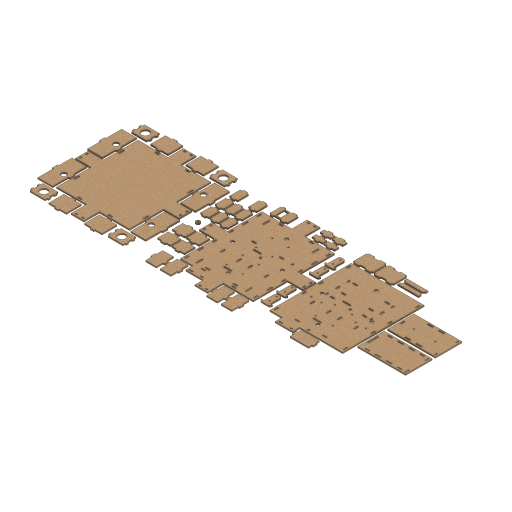
# Autodesk Inventor part: Pieza1
Saved by Autodesk Inventor 2024 (Build 280153000, 153)
## iProperties
Created: 2023-11-21
Part Number: Pieza1
Material: MDF Tablero de fibras de densidad media
Document SubType Name: Modeling
Designer: marco
Density: 0.8 g/cm^3
Appearance: Cartón - Ondulado
Author: marco
Autodesk Inventor part; units mm, degrees
(part 1 of 2)
ref_plane "YZ Plane" through (0, 0, 0) normal (1, 0, 0) x (0, 1, 0)
ref_plane "XZ Plane" through (0, 0, 0) normal (0, 1, 0) x (-1, 0, 0)
ref_plane "XY Plane" through (0, 0, 0) normal (0, 0, 1) x (1, 0, 0)
sketch "Boceto1" plane through (0, 0, 0) normal (0, 1, 0) x (-1, 0, 0)
  line L0 (397.5, 103.5) -> (397.5, 108.5)
  line L1 (397.5, 108.5) -> (400.5, 108.5)
  line L2 (400.5, 108.5) -> (400.5, 113.5)
  line L3 (400.5, 113.5) -> (397.5, 113.5)
  line L4 (397.5, 113.5) -> (397.5, 123.5)
  line L5 (397.5, 123.5) -> (400.5, 123.5)
  line L6 (400.5, 123.5) -> (400.5, 128.5)
  line L7 (400.5, 128.5) -> (397.5, 128.5)
  line L8 (397.5, 128.5) -> (397.5, 133.5)
  line L9 (397.5, 133.5) -> (362.5, 133.5)
  line L10 (362.5, 133.5) -> (362.5, 128.5)
  line L11 (362.5, 128.5) -> (359.5, 128.5)
  line L12 (359.5, 128.5) -> (359.5, 123.5)
  line L13 (359.5, 123.5) -> (362.5, 123.5)
  line L14 (362.5, 123.5) -> (362.5, 113.5)
  line L15 (362.5, 113.5) -> (359.5, 113.5)
  line L16 (359.5, 113.5) -> (359.5, 108.5)
  line L17 (359.5, 108.5) -> (362.5, 108.5)
  line L18 (362.5, 108.5) -> (362.5, 103.5)
  line L19 (362.5, 103.5) -> (397.5, 103.5)
  line L20 (180.5, 133.5) -> (180.5, 128.5)
  line L21 (180.5, 128.5) -> (177.5, 128.5)
  line L22 (177.5, 128.5) -> (177.5, 123.5)
  line L23 (177.5, 123.5) -> (180.5, 123.5)
  line L24 (180.5, 123.5) -> (180.5, 113.5)
  line L25 (180.5, 113.5) -> (177.5, 113.5)
  line L26 (177.5, 113.5) -> (177.5, 108.5)
  line L27 (177.5, 108.5) -> (180.5, 108.5)
  line L28 (180.5, 108.5) -> (180.5, 103.5)
  line L29 (180.5, 103.5) -> (215.5, 103.5)
  line L30 (215.5, 103.5) -> (215.5, 108.5)
  line L31 (215.5, 108.5) -> (218.5, 108.5)
  line L32 (218.5, 108.5) -> (218.5, 113.5)
  line L33 (218.5, 113.5) -> (215.5, 113.5)
  line L34 (215.5, 113.5) -> (215.5, 123.5)
  line L35 (215.5, 123.5) -> (218.5, 123.5)
  line L36 (218.5, 123.5) -> (218.5, 128.5)
  line L37 (218.5, 128.5) -> (215.5, 128.5)
  line L38 (215.5, 128.5) -> (215.5, 133.5)
  line L39 (215.5, 133.5) -> (180.5, 133.5)
  line L40 (329, -92) -> (320, -92)
  line L41 (320, -92) -> (320, -89)
  line L42 (320, -89) -> (329, -89)
  line L43 (329, -89) -> (329, -92)
  line L44 (371, 58) -> (368, 58)
  line L45 (368, 58) -> (368, 46)
  line L46 (368, 46) -> (371, 46)
  line L47 (371, 46) -> (371, 58)
  line L48 (320, 92) -> (329, 92)
  line L49 (329, 92) -> (329, 89)
  line L50 (329, 89) -> (320, 89)
  line L51 (320, 89) -> (320, 92)
  line L52 (371, -46) -> (368, -46)
  line L53 (368, -46) -> (368, -58)
  line L54 (368, -58) -> (371, -58)
  line L55 (371, -58) -> (371, -46)
  line L56 (207, -46) -> (210, -46)
  line L57 (210, -46) -> (210, -58)
  line L58 (210, -58) -> (207, -58)
  line L59 (207, -58) -> (207, -46)
  line L60 (174, -10) -> (171, -10)
  line L61 (171, -10) -> (171, -5)
  line L62 (171, -5) -> (174, -5)
  line L63 (174, -5) -> (174, -10)
  line L64 (207, 46) -> (210, 46)
  line L65 (210, 46) -> (210, 58)
  line L66 (210, 58) -> (207, 58)
  line L67 (207, 58) -> (207, 46)
  line L68 (258, -92) -> (249, -92)
  line L69 (249, -92) -> (249, -89)
  line L70 (249, -89) -> (258, -89)
  line L71 (258, -89) -> (258, -92)
  line L72 (279, -128) -> (279, -125)
  line L73 (279, -125) -> (284, -125)
  line L74 (284, -125) -> (284, -128)
  line L75 (284, -128) -> (279, -128)
  line L76 (299, 125) -> (294, 125)
  line L77 (294, 125) -> (294, 128)
  line L78 (294, 128) -> (299, 128)
  line L79 (299, 128) -> (299, 125)
  line L80 (284, 128) -> (279, 128)
  line L81 (279, 128) -> (279, 125)
  line L82 (279, 125) -> (284, 125)
  line L83 (284, 125) -> (284, 128)
  line L84 (404, -10) -> (404, -5)
  line L85 (404, -5) -> (407, -5)
  line L86 (407, -5) -> (407, -10)
  line L87 (407, -10) -> (404, -10)
  line L88 (404, 5) -> (404, 10)
  line L89 (404, 10) -> (407, 10)
  line L90 (407, 10) -> (407, 5)
  line L91 (407, 5) -> (404, 5)
  line L92 (299, -125) -> (294, -125)
  line L93 (294, -125) -> (294, -128)
  line L94 (294, -128) -> (299, -128)
  line L95 (299, -128) -> (299, -125)
  line L96 (174, 10) -> (174, 5)
  line L97 (174, 5) -> (171, 5)
  line L98 (171, 5) -> (171, 10)
  line L99 (171, 10) -> (174, 10)
  line L100 (415, -49) -> (418, -49)
  line L101 (418, -49) -> (418, -61)
  line L102 (418, -61) -> (415, -61)
  line L103 (415, -61) -> (415, -98)
  line L104 (415, -98) -> (380, -98)
  line L105 (380, -98) -> (380, -61)
  line L106 (380, -61) -> (377, -61)
  line L107 (377, -61) -> (377, -49)
  line L108 (377, -49) -> (380, -49)
  line L109 (380, -49) -> (380, -18)
  line L110 (380, -18) -> (415, -18)
  line L111 (415, -18) -> (415, -49)
  line L112 (377, 49) -> (377, 61)
  line L113 (377, 61) -> (380, 61)
  line L114 (380, 61) -> (380, 98)
  line L115 (380, 98) -> (415, 98)
  line L116 (415, 98) -> (415, 61)
  line L117 (415, 61) -> (418, 61)
  line L118 (418, 61) -> (418, 49)
  line L119 (418, 49) -> (415, 49)
  line L120 (415, 49) -> (415, 18)
  line L121 (415, 18) -> (380, 18)
  line L122 (380, 18) -> (380, 49)
  line L123 (380, 49) -> (377, 49)
  line L124 (163, 98) -> (198, 98)
  line L125 (198, 98) -> (198, 61)
  line L126 (198, 61) -> (201, 61)
  line L127 (201, 61) -> (201, 49)
  line L128 (201, 49) -> (198, 49)
  line L129 (198, 49) -> (198, 18)
  line L130 (198, 18) -> (163, 18)
  line L131 (163, 18) -> (163, 49)
  line L132 (163, 49) -> (160, 49)
  line L133 (160, 49) -> (160, 61)
  line L134 (160, 61) -> (163, 61)
  line L135 (163, 61) -> (163, 98)
  line L136 (258, 92) -> (249, 92)
  line L137 (249, 92) -> (249, 89)
  line L138 (249, 89) -> (258, 89)
  line L139 (258, 89) -> (258, 92)
  line L140 (310, 101) -> (310, 136)
  line L141 (310, 136) -> (326, 136)
  line L142 (326, 136) -> (326, 139)
  line L143 (326, 139) -> (335, 139)
  line L144 (335, 139) -> (335, 136)
  line L145 (335, 136) -> (351, 136)
  line L146 (351, 136) -> (351, 101)
  line L147 (351, 101) -> (335, 101)
  line L148 (335, 101) -> (335, 98)
  line L149 (335, 98) -> (326, 98)
  line L150 (326, 98) -> (326, 101)
  line L151 (326, 101) -> (310, 101)
  line L152 (310, -136) -> (310, -101)
  line L153 (310, -101) -> (326, -101)
  line L154 (326, -101) -> (326, -98)
  line L155 (326, -98) -> (335, -98)
  line L156 (335, -98) -> (335, -101)
  line L157 (335, -101) -> (351, -101)
  line L158 (351, -101) -> (351, -136)
  line L159 (351, -136) -> (335, -136)
  line L160 (335, -136) -> (335, -139)
  line L161 (335, -139) -> (326, -139)
  line L162 (326, -139) -> (326, -136)
  line L163 (326, -136) -> (310, -136)
  line L164 (362.5, -133.5) -> (397.5, -133.5)
  line L165 (397.5, -133.5) -> (397.5, -128.5)
  line L166 (397.5, -128.5) -> (400.5, -128.5)
  line L167 (400.5, -128.5) -> (400.5, -123.5)
  line L168 (400.5, -123.5) -> (397.5, -123.5)
  line L169 (397.5, -123.5) -> (397.5, -113.5)
  line L170 (397.5, -113.5) -> (400.5, -113.5)
  line L171 (400.5, -113.5) -> (400.5, -108.5)
  line L172 (400.5, -108.5) -> (397.5, -108.5)
  line L173 (397.5, -108.5) -> (397.5, -103.5)
  line L174 (397.5, -103.5) -> (362.5, -103.5)
  line L175 (362.5, -103.5) -> (362.5, -108.5)
  line L176 (362.5, -108.5) -> (359.5, -108.5)
  line L177 (359.5, -108.5) -> (359.5, -113.5)
  line L178 (359.5, -113.5) -> (362.5, -113.5)
  line L179 (362.5, -113.5) -> (362.5, -123.5)
  line L180 (362.5, -123.5) -> (359.5, -123.5)
  line L181 (359.5, -123.5) -> (359.5, -128.5)
  line L182 (359.5, -128.5) -> (362.5, -128.5)
  line L183 (362.5, -128.5) -> (362.5, -133.5)
  line L184 (177.5, -123.5) -> (177.5, -128.5)
  line L185 (177.5, -128.5) -> (180.5, -128.5)
  line L186 (180.5, -128.5) -> (180.5, -133.5)
  line L187 (180.5, -133.5) -> (215.5, -133.5)
  line L188 (215.5, -133.5) -> (215.5, -128.5)
  line L189 (215.5, -128.5) -> (218.5, -128.5)
  line L190 (218.5, -128.5) -> (218.5, -123.5)
  line L191 (218.5, -123.5) -> (215.5, -123.5)
  line L192 (215.5, -123.5) -> (215.5, -113.5)
  line L193 (215.5, -113.5) -> (218.5, -113.5)
  line L194 (218.5, -113.5) -> (218.5, -108.5)
  line L195 (218.5, -108.5) -> (215.5, -108.5)
  line L196 (215.5, -108.5) -> (215.5, -103.5)
  line L197 (215.5, -103.5) -> (180.5, -103.5)
  line L198 (180.5, -103.5) -> (180.5, -108.5)
  line L199 (180.5, -108.5) -> (177.5, -108.5)
  line L200 (177.5, -108.5) -> (177.5, -113.5)
  line L201 (177.5, -113.5) -> (180.5, -113.5)
  line L202 (180.5, -113.5) -> (180.5, -123.5)
  line L203 (180.5, -123.5) -> (177.5, -123.5)
  line L204 (138.7318, -1.5139) -> (136.2318, -1.5139)
  line L205 (136.2318, -1.5139) -> (136.2318, 1.4861)
  line L206 (136.2318, 1.4861) -> (141.2318, 1.4861)
  line L207 (141.2318, 1.4861) -> (141.2318, -1.5139)
  line L208 (141.2318, -1.5139) -> (138.7318, -1.5139)
  line L209 (-20.6092, 99.402) -> (-20.6092, 114.402)
  line L210 (-20.6092, 114.402) -> (-17.6092, 114.402)
  line L211 (-17.6092, 114.402) -> (-17.6092, 124.402)
  line L212 (-17.6092, 124.402) -> (-20.6092, 124.402)
  line L213 (-20.6092, 124.402) -> (-20.6092, 139.402)
  line L214 (-20.6092, 139.402) -> (-45.6092, 139.402)
  line L215 (-45.6092, 139.402) -> (-45.6092, 124.402)
  line L216 (-45.6092, 124.402) -> (-48.6092, 124.402)
  line L217 (-48.6092, 124.402) -> (-48.6092, 114.402)
  line L218 (-48.6092, 114.402) -> (-45.6092, 114.402)
  line L219 (-45.6092, 114.402) -> (-45.6092, 99.402)
  line L220 (-45.6092, 99.402) -> (-20.6092, 99.402)
  line L221 (45.6946, -98.4202) -> (36.6946, -98.4202)
  line L222 (36.6946, -98.4202) -> (36.6946, -101.4202)
  line L223 (36.6946, -101.4202) -> (31.6946, -101.4202)
  line L224 (31.6946, -101.4202) -> (31.6946, -126.4202)
  line L225 (31.6946, -126.4202) -> (36.6946, -126.4202)
  line L226 (36.6946, -126.4202) -> (36.6946, -129.4202)
  line L227 (36.6946, -129.4202) -> (45.6946, -129.4202)
  line L228 (45.6946, -129.4202) -> (45.6946, -126.4202)
  line L229 (45.6946, -126.4202) -> (63.1946, -126.4202)
  line L230 (63.1946, -126.4202) -> (63.1946, -129.4202)
  line L231 (63.1946, -129.4202) -> (69.1946, -129.4202)
  line L232 (69.1946, -98.4202) -> (63.1946, -98.4202)
  line L233 (63.1946, -98.4202) -> (63.1946, -101.4202)
  line L234 (63.1946, -101.4202) -> (45.6946, -101.4202)
  line L235 (45.6946, -101.4202) -> (45.6946, -98.4202)
  line L236 (-54.5593, 99.402) -> (-54.5593, 114.402)
  line L237 (-54.5593, 114.402) -> (-51.5593, 114.402)
  line L238 (-51.5593, 114.402) -> (-51.5593, 124.402)
  line L239 (-51.5593, 124.402) -> (-54.5593, 124.402)
  line L240 (-54.5593, 124.402) -> (-54.5593, 139.402)
  line L241 (-54.5593, 139.402) -> (-79.5593, 139.402)
  line L242 (-79.5593, 139.402) -> (-79.5593, 124.402)
  line L243 (-79.5593, 124.402) -> (-82.5593, 124.402)
  line L244 (-82.5593, 124.402) -> (-82.5593, 114.402)
  line L245 (-82.5593, 114.402) -> (-79.5593, 114.402)
  line L246 (-79.5593, 114.402) -> (-79.5593, 99.402)
  line L247 (-79.5593, 99.402) -> (-54.5593, 99.402)
  line L248 (121.6406, 99.402) -> (121.6406, 114.402)
  line L249 (121.6406, 114.402) -> (124.6406, 114.402)
  line L250 (124.6406, 114.402) -> (124.6406, 124.402)
  line L251 (124.6406, 124.402) -> (121.6406, 124.402)
  line L252 (121.6406, 124.402) -> (121.6406, 139.402)
  line L253 (121.6406, 139.402) -> (96.6406, 139.402)
  line L254 (96.6406, 139.402) -> (96.6406, 124.402)
  line L255 (96.6406, 124.402) -> (93.6406, 124.402)
  line L256 (93.6406, 124.402) -> (93.6406, 114.402)
  line L257 (93.6406, 114.402) -> (96.6406, 114.402)
  line L258 (96.6406, 114.402) -> (96.6406, 99.402)
  line L259 (96.6406, 99.402) -> (121.6406, 99.402)
  line L260 (87.6406, 99.402) -> (87.6406, 114.402)
  line L261 (87.6406, 114.402) -> (90.6406, 114.402)
  line L262 (90.6406, 114.402) -> (90.6406, 124.402)
  line L263 (90.6406, 124.402) -> (87.6406, 124.402)
  line L264 (87.6406, 124.402) -> (87.6406, 139.402)
  line L265 (87.6406, 139.402) -> (62.6406, 139.402)
  line L266 (62.6406, 139.402) -> (62.6406, 124.402)
  line L267 (62.6406, 124.402) -> (59.6406, 124.402)
  line L268 (59.6406, 124.402) -> (59.6406, 114.402)
  line L269 (59.6406, 114.402) -> (62.6406, 114.402)
  line L270 (62.6406, 114.402) -> (62.6406, 99.402)
  line L271 (62.6406, 99.402) -> (87.6406, 99.402)
  line L272 (-24.9127, -131.1401) -> (-32.4127, -131.1401)
  line L273 (-32.4127, -131.1401) -> (-32.4127, -134.1401)
  line L274 (-32.4127, -134.1401) -> (-42.4127, -134.1401)
  line L275 (-42.4127, -134.1401) -> (-42.4127, -131.1401)
  line L276 (-42.4127, -131.1401) -> (-49.9127, -131.1401)
  line L277 (-49.9127, -131.1401) -> (-49.9127, -121.1401)
  line L278 (-49.9127, -121.1401) -> (-42.4127, -121.1401)
  line L279 (-42.4127, -121.1401) -> (-42.4127, -118.1401)
  line L280 (-42.4127, -118.1401) -> (-32.4127, -118.1401)
  line L281 (-32.4127, -118.1401) -> (-32.4127, -121.1401)
  line L282 (-32.4127, -121.1401) -> (-24.9127, -121.1401)
  line L283 (-24.9127, -121.1401) -> (-24.9127, -131.1401)
  line L284 (-387.9327, 9.6476) -> (-397.9327, 9.6476)
  line L285 (-397.9327, 9.6476) -> (-397.9327, 6.6476)
  line L286 (-397.9327, 6.6476) -> (-387.9327, 6.6476)
  line L287 (-387.9327, 6.6476) -> (-387.9327, 9.6476)
  line L288 (-411.4327, 3.6476) -> (-299.4327, 3.6476)
  line L289 (-299.4327, 3.6476) -> (-299.4327, 65.6476)
  line L290 (-299.4327, 65.6476) -> (-411.4327, 65.6476)
  line L291 (-411.4327, 65.6476) -> (-411.4327, 3.6476)
  line L292 (-322.9327, 59.6476) -> (-322.9327, 62.6476)
  line L293 (-322.9327, 62.6476) -> (-312.9327, 62.6476)
  line L294 (-312.9327, 62.6476) -> (-312.9327, 59.6476)
  line L295 (-312.9327, 59.6476) -> (-322.9327, 59.6476)
  line L296 (-322.9327, 9.6476) -> (-322.9327, 6.6476)
  line L297 (-322.9327, 6.6476) -> (-312.9327, 6.6476)
  line L298 (-312.9327, 6.6476) -> (-312.9327, 9.6476)
  line L299 (-312.9327, 9.6476) -> (-322.9327, 9.6476)
  line L300 (-312.9327, 9.6476) -> (-322.9327, 9.6476)
  line L301 (-322.9327, 9.6476) -> (-322.9327, 6.6476)
  line L302 (-322.9327, 6.6476) -> (-312.9327, 6.6476)
  line L303 (-312.9327, 6.6476) -> (-312.9327, 9.6476)
  line L304 (-397.9327, 59.6476) -> (-387.9327, 59.6476)
  line L305 (-387.9327, 59.6476) -> (-387.9327, 62.6476)
  line L306 (-387.9327, 62.6476) -> (-397.9327, 62.6476)
  line L307 (-397.9327, 62.6476) -> (-397.9327, 59.6476)
  line L308 (-335.9327, 6.6476) -> (-348.9327, 6.6476)
  line L309 (-348.9327, 6.6476) -> (-348.9327, 9.6476)
  line L310 (-348.9327, 9.6476) -> (-335.9327, 9.6476)
  line L311 (-335.9327, 9.6476) -> (-335.9327, 6.6476)
  line L312 (-361.9327, 6.6476) -> (-374.9327, 6.6476)
  line L313 (-374.9327, 6.6476) -> (-374.9327, 9.6476)
  line L314 (-374.9327, 9.6476) -> (-361.9327, 9.6476)
  line L315 (-361.9327, 9.6476) -> (-361.9327, 6.6476)
  line L316 (-335.9327, 62.6476) -> (-335.9327, 59.6476)
  line L317 (-335.9327, 59.6476) -> (-348.9327, 59.6476)
  line L318 (-348.9327, 59.6476) -> (-348.9327, 62.6476)
  line L319 (-348.9327, 62.6476) -> (-335.9327, 62.6476)
  line L320 (-361.9327, 62.6476) -> (-361.9327, 59.6476)
  line L321 (-361.9327, 59.6476) -> (-374.9327, 59.6476)
  line L322 (-374.9327, 59.6476) -> (-374.9327, 62.6476)
  line L323 (-374.9327, 62.6476) -> (-361.9327, 62.6476)
  line L324 (-60.4127, -134.1401) -> (-60.4127, -131.1401)
  line L325 (-60.4127, -131.1401) -> (-52.9127, -131.1401)
  line L326 (-52.9127, -131.1401) -> (-52.9127, -121.1401)
  line L327 (-52.9127, -121.1401) -> (-60.4127, -121.1401)
  line L328 (-60.4127, -121.1401) -> (-60.4127, -118.1401)
  line L329 (-60.4127, -118.1401) -> (-70.4127, -118.1401)
  line L330 (-70.4127, -118.1401) -> (-70.4127, -121.1401)
  line L331 (-70.4127, -121.1401) -> (-77.9127, -121.1401)
  line L332 (-77.9127, -121.1401) -> (-77.9127, -131.1401)
  line L333 (-77.9127, -131.1401) -> (-70.4127, -131.1401)
  line L334 (-70.4127, -131.1401) -> (-70.4127, -134.1401)
  line L335 (-70.4127, -134.1401) -> (-60.4127, -134.1401)
  line L336 (-77.9127, -102.1401) -> (-77.9127, -112.1401)
  line L337 (-77.9127, -112.1401) -> (-70.4127, -112.1401)
  line L338 (-70.4127, -112.1401) -> (-70.4127, -115.1401)
  line L339 (-70.4127, -115.1401) -> (-60.4127, -115.1401)
  line L340 (-60.4127, -115.1401) -> (-60.4127, -112.1401)
  line L341 (-60.4127, -112.1401) -> (-52.9127, -112.1401)
  line L342 (-52.9127, -112.1401) -> (-52.9127, -102.1401)
  line L343 (-52.9127, -102.1401) -> (-60.4127, -102.1401)
  line L344 (-60.4127, -102.1401) -> (-60.4127, -99.1401)
  line L345 (-60.4127, -99.1401) -> (-70.4127, -99.1401)
  line L346 (-70.4127, -99.1401) -> (-70.4127, -102.1401)
  line L347 (-70.4127, -102.1401) -> (-77.9127, -102.1401)
  line L348 (-32.4127, -115.1401) -> (-32.4127, -112.1401)
  line L349 (-32.4127, -112.1401) -> (-24.9127, -112.1401)
  line L350 (-24.9127, -112.1401) -> (-24.9127, -102.1401)
  line L351 (-24.9127, -102.1401) -> (-32.4127, -102.1401)
  line L352 (-32.4127, -102.1401) -> (-32.4127, -99.1401)
  line L353 (-32.4127, -99.1401) -> (-42.4127, -99.1401)
  line L354 (-42.4127, -99.1401) -> (-42.4127, -102.1401)
  line L355 (-42.4127, -102.1401) -> (-49.9127, -102.1401)
  line L356 (-49.9127, -102.1401) -> (-49.9127, -112.1401)
  line L357 (-49.9127, -112.1401) -> (-42.4127, -112.1401)
  line L358 (-42.4127, -112.1401) -> (-42.4127, -115.1401)
  line L359 (-42.4127, -115.1401) -> (-32.4127, -115.1401)
  line L360 (-186.5302, -131.9693) -> (-186.5302, -134.9693)
  line L361 (-186.5302, -134.9693) -> (-173.5302, -134.9693)
  line L362 (-173.5302, -134.9693) -> (-173.5302, -131.9693)
  line L363 (-173.5302, -131.9693) -> (-170.5302, -131.9693)
  line L364 (-170.5302, -131.9693) -> (-170.5302, -101.9693)
  line L365 (-170.5302, -101.9693) -> (-173.5302, -101.9693)
  line L366 (-173.5302, -101.9693) -> (-173.5302, -98.9693)
  line L367 (-173.5302, -98.9693) -> (-186.5302, -98.9693)
  line L368 (-186.5302, -98.9693) -> (-186.5302, -101.9693)
  line L369 (-186.5302, -101.9693) -> (-199.5302, -101.9693)
  line L370 (-199.5302, -101.9693) -> (-199.5302, -98.9693)
  line L371 (-199.5302, -98.9693) -> (-212.5302, -98.9693)
  line L372 (-212.5302, -98.9693) -> (-212.5302, -101.9693)
  line L373 (-212.5302, -101.9693) -> (-215.5302, -101.9693)
  line L374 (-215.5302, -101.9693) -> (-215.5302, -131.9693)
  line L375 (-215.5302, -131.9693) -> (-212.5302, -131.9693)
  line L376 (-212.5302, -131.9693) -> (-212.5302, -134.9693)
  line L377 (-212.5302, -134.9693) -> (-199.5302, -134.9693)
  line L378 (-199.5302, -134.9693) -> (-199.5302, -131.9693)
  line L379 (-199.5302, -131.9693) -> (-186.5302, -131.9693)
  line L380 (-138.5302, -131.9693) -> (-138.5302, -134.9693)
  line L381 (-138.5302, -134.9693) -> (-125.5302, -134.9693)
  line L382 (-125.5302, -134.9693) -> (-125.5302, -131.9693)
  line L383 (-125.5302, -131.9693) -> (-122.5302, -131.9693)
  line L384 (-122.5302, -131.9693) -> (-122.5302, -101.9693)
  line L385 (-122.5302, -101.9693) -> (-125.5302, -101.9693)
  line L386 (-125.5302, -101.9693) -> (-125.5302, -98.9693)
  line L387 (-125.5302, -98.9693) -> (-138.5302, -98.9693)
  line L388 (-138.5302, -98.9693) -> (-138.5302, -101.9693)
  line L389 (-138.5302, -101.9693) -> (-151.5302, -101.9693)
  line L390 (-151.5302, -101.9693) -> (-151.5302, -98.9693)
  line L391 (-151.5302, -98.9693) -> (-164.5302, -98.9693)
  line L392 (-164.5302, -98.9693) -> (-164.5302, -101.9693)
  line L393 (-164.5302, -101.9693) -> (-167.5302, -101.9693)
  line L394 (-167.5302, -101.9693) -> (-167.5302, -131.9693)
  line L395 (-167.5302, -131.9693) -> (-164.5302, -131.9693)
  line L396 (-164.5302, -131.9693) -> (-164.5302, -134.9693)
  line L397 (-164.5302, -134.9693) -> (-151.5302, -134.9693)
  line L398 (-151.5302, -134.9693) -> (-151.5302, -131.9693)
  line L399 (-151.5302, -131.9693) -> (-138.5302, -131.9693)
  line L400 (-243.5117, 124.2705) -> (-200.5117, 124.2705)
  line L401 (-200.5117, 124.2705) -> (-200.5117, 116.2705)
  line L402 (-200.5117, 116.2705) -> (-197.5117, 116.2705)
  line L403 (-197.5117, 116.2705) -> (-197.5117, 107.2705)
  line L404 (-197.5117, 107.2705) -> (-200.5117, 107.2705)
  line L405 (-200.5117, 107.2705) -> (-200.5117, 99.2705)
  line L406 (-200.5117, 99.2705) -> (-243.5117, 99.2705)
  line L407 (-243.5117, 99.2705) -> (-243.5117, 107.2705)
  line L408 (-243.5117, 107.2705) -> (-246.5117, 107.2705)
  line L409 (-246.5117, 107.2705) -> (-246.5117, 116.2705)
  line L410 (-246.5117, 116.2705) -> (-243.5117, 116.2705)
  line L411 (-243.5117, 116.2705) -> (-243.5117, 124.2705)
  line L412 (-266.5396, -115.5839) -> (-266.5396, -112.5839)
  line L413 (-266.5396, -112.5839) -> (-269.5396, -112.5839)
  line L414 (-269.5396, -112.5839) -> (-269.5396, -106.5839)
  line L415 (-269.5396, -106.5839) -> (-266.5396, -106.5839)
  line L416 (-266.5396, -106.5839) -> (-223.5396, -106.5839)
  line L417 (-223.5396, -106.5839) -> (-220.5396, -106.5839)
  line L418 (-220.5396, -106.5839) -> (-220.5396, -112.5839)
  line L419 (-220.5396, -112.5839) -> (-223.5396, -112.5839)
  line L420 (-223.5396, -112.5839) -> (-223.5396, -115.5839)
  line L421 (-223.5396, -115.5839) -> (-266.5396, -115.5839)
  line L422 (-223.5396, -119.5483) -> (-266.5396, -119.5483)
  line L423 (-266.5396, -119.5483) -> (-266.5396, -122.5483)
  line L424 (-266.5396, -122.5483) -> (-269.5396, -122.5483)
  line L425 (-269.5396, -122.5483) -> (-269.5396, -128.5483)
  line L426 (-269.5396, -128.5483) -> (-266.5396, -128.5483)
  line L427 (-266.5396, -128.5483) -> (-223.5396, -128.5483)
  line L428 (-223.5396, -128.5483) -> (-220.5396, -128.5483)
  line L429 (-220.5396, -128.5483) -> (-220.5396, -122.5483)
  line L430 (-220.5396, -122.5483) -> (-223.5396, -122.5483)
  line L431 (-223.5396, -122.5483) -> (-223.5396, -119.5483)
  line L432 (-408.4327, 6.6476) -> (-405.4327, 6.6476)
  line L433 (-405.4327, 15.6476) -> (-408.4327, 15.6476)
  line L434 (-405.4327, 62.6476) -> (-405.4327, 53.6476)
  line L435 (-405.4327, 53.6476) -> (-408.4327, 53.6476)
  line L436 (-408.4327, 53.6476) -> (-408.4327, 62.6476)
  line L437 (-408.4327, 62.6476) -> (-405.4327, 62.6476)
  line L438 (61.4446, -123.4202) -> (61.4446, -104.4202)
  line L439 (61.4446, -104.4202) -> (50.4446, -104.4202)
  line L440 (50.4446, -104.4202) -> (50.4446, -123.4202)
  line L441 (50.4446, -123.4202) -> (61.4446, -123.4202)
  line L442 (-335.9327, -62.749) -> (-348.9327, -62.749)
  line L443 (-348.9327, -62.749) -> (-348.9327, -59.749)
  line L444 (-348.9327, -59.749) -> (-335.9327, -59.749)
  line L445 (-335.9327, -59.749) -> (-335.9327, -62.749)
  line L446 (-374.9327, -59.749) -> (-361.9327, -59.749)
  line L447 (-361.9327, -59.749) -> (-361.9327, -62.749)
  line L448 (-361.9327, -62.749) -> (-374.9327, -62.749)
  line L449 (-374.9327, -62.749) -> (-374.9327, -59.749)
  line L450 (-374.9327, -9.749) -> (-361.9327, -9.749)
  line L451 (-361.9327, -9.749) -> (-361.9327, -6.749)
  line L452 (-361.9327, -6.749) -> (-374.9327, -6.749)
  line L453 (-374.9327, -6.749) -> (-374.9327, -9.749)
  line L454 (-299.4327, -65.749) -> (-411.4327, -65.749)
  line L455 (-411.4327, -65.749) -> (-411.4327, -3.749)
  line L456 (-411.4327, -3.749) -> (-299.4327, -3.749)
  line L457 (-299.4327, -3.749) -> (-299.4327, -65.749)
  line L458 (-335.9327, -9.749) -> (-348.9327, -9.749)
  line L459 (-348.9327, -9.749) -> (-348.9327, -6.749)
  line L460 (-348.9327, -6.749) -> (-335.9327, -6.749)
  line L461 (-335.9327, -6.749) -> (-335.9327, -9.749)
  line L462 (-305.4327, 47.1476) -> (-302.4327, 47.1476)
  line L463 (-302.4327, 47.1476) -> (-302.4327, 22.1476)
  line L464 (-302.4327, 22.1476) -> (-305.4327, 22.1476)
  line L465 (-305.4327, 22.1476) -> (-305.4327, 47.1476)
  line L466 (-405.4327, -6.749) -> (-408.4327, -6.749)
  line L467 (-408.4327, -6.749) -> (-408.4327, -12.749)
  line L468 (-408.4327, -12.749) -> (-405.4327, -12.749)
  line L469 (-405.4327, -12.749) -> (-405.4327, -6.749)
  line L470 (-302.4327, -39.249) -> (-305.4327, -39.249)
  line L471 (-305.4327, -39.249) -> (-305.4327, -30.249)
  line L472 (-305.4327, -30.249) -> (-302.4327, -30.249)
  line L473 (-302.4327, -30.249) -> (-302.4327, -39.249)
  line L474 (304, -95) -> (374, -95)
  line L475 (374, -95) -> (374, -15)
  line L476 (374, -15) -> (410, -15)
  line L477 (410, -15) -> (410, 15)
  line L478 (410, 15) -> (374, 15)
  line L479 (374, 15) -> (374, 95)
  line L480 (374, 95) -> (304, 95)
  line L481 (304, 95) -> (304, 131)
  line L482 (304, 131) -> (274, 131)
  line L483 (274, 131) -> (274, 95)
  line L484 (274, 95) -> (204, 95)
  line L485 (204, 95) -> (204, 15)
  line L486 (274, -95) -> (204, -95)
  line L487 (204, -95) -> (204, -15)
  line L488 (204, -15) -> (168, -15)
  line L489 (201, -61) -> (198, -61)
  line L490 (198, -61) -> (198, -98)
  line L491 (198, -98) -> (163, -98)
  line L492 (163, -98) -> (163, -61)
  line L493 (163, -61) -> (160, -61)
  line L494 (160, -61) -> (160, -49)
  line L495 (140, -86) -> (140, -89)
  line L496 (140, -89) -> (135, -89)
  line L497 (135, -89) -> (135, -114)
  line L498 (135, -114) -> (140, -114)
  line L499 (140, -114) -> (140, -117)
  line L500 (140, -86) -> (149, -86)
  line L501 (149, -86) -> (149, -89)
  line L502 (149, -89) -> (154, -89)
  line L503 (154, -89) -> (154, -114)
  line L504 (154, -114) -> (149, -114)
  line L505 (149, -114) -> (149, -117)
  line L506 (149, -117) -> (140, -117)
  line L507 (243, 98) -> (243, 101)
  line L508 (243, 101) -> (227, 101)
  line L509 (227, 101) -> (227, 136)
  line L510 (227, 136) -> (243, 136)
  line L511 (243, 136) -> (243, 139)
  line L512 (243, 139) -> (252, 139)
  line L513 (252, 139) -> (252, 136)
  line L514 (252, 136) -> (268, 136)
  line L515 (268, 101) -> (252, 101)
  line L516 (252, 101) -> (252, 98)
  line L517 (252, 98) -> (243, 98)
  line L518 (268, -136) -> (252, -136)
  line L519 (252, -136) -> (252, -139)
  line L520 (252, -139) -> (243, -139)
  line L521 (243, -139) -> (243, -136)
  line L522 (243, -136) -> (227, -136)
  line L523 (227, -136) -> (227, -101)
  line L524 (227, -101) -> (243, -101)
  line L525 (243, -101) -> (243, -98)
  line L526 (153.241, 46) -> (143.241, 46)
  line L527 (143.241, 46) -> (143.241, 49)
  line L528 (143.241, 49) -> (133.241, 49)
  line L529 (133.241, 49) -> (133.241, 46)
  line L530 (133.241, 46) -> (123.241, 46)
  line L531 (123.241, 46) -> (123.241, 21)
  line L532 (123.241, 21) -> (133.241, 21)
  line L533 (133.241, 21) -> (133.241, 18)
  line L534 (133.241, 18) -> (143.241, 18)
  line L535 (143.241, 18) -> (143.241, 21)
  line L536 (143.241, 21) -> (153.241, 21)
  line L537 (153.241, 21) -> (153.241, 46)
  line L538 (96, -117) -> (105, -117)
  line L539 (105, -117) -> (105, -114)
  line L540 (105, -114) -> (110, -114)
  line L541 (110, -114) -> (110, -89)
  line L542 (96, -117) -> (96, -114)
  line L543 (96, -114) -> (91, -114)
  line L544 (91, -114) -> (91, -89)
  line L545 (91, -89) -> (96, -89)
  line L546 (96, -89) -> (96, -86)
  line L547 (96, -86) -> (105, -86)
  line L548 (105, -86) -> (105, -89)
  line L549 (105, -89) -> (110, -89)
  line L550 (140, -52) -> (149, -52)
  line L551 (149, -52) -> (149, -55)
  line L552 (149, -55) -> (154, -55)
  line L553 (140, -83) -> (149, -83)
  line L554 (149, -83) -> (149, -80)
  line L555 (149, -80) -> (154, -80)
  line L556 (154, -80) -> (154, -55)
  line L557 (140, -52) -> (140, -55)
  line L558 (140, -55) -> (135, -55)
  line L559 (135, -55) -> (135, -80)
  line L560 (135, -80) -> (140, -80)
  line L561 (140, -80) -> (140, -83)
  line L562 (118, -52) -> (127, -52)
  line L563 (127, -52) -> (127, -55)
  line L564 (127, -55) -> (132, -55)
  line L565 (132, -55) -> (132, -80)
  line L566 (132, -80) -> (127, -80)
  line L567 (127, -80) -> (127, -83)
  line L568 (127, -83) -> (118, -83)
  line L569 (118, -52) -> (118, -55)
  line L570 (118, -55) -> (113, -55)
  line L571 (113, -55) -> (113, -80)
  line L572 (113, -80) -> (118, -80)
  line L573 (118, -80) -> (118, -83)
  line L574 (96, -83) -> (105, -83)
  line L575 (105, -83) -> (105, -80)
  line L576 (105, -80) -> (110, -80)
  line L577 (110, -80) -> (110, -55)
  line L578 (96, -52) -> (96, -55)
  line L579 (96, -55) -> (91, -55)
  line L580 (91, -55) -> (91, -80)
  line L581 (91, -80) -> (96, -80)
  line L582 (96, -80) -> (96, -83)
  line L583 (96, -52) -> (105, -52)
  line L584 (105, -52) -> (105, -55)
  line L585 (105, -55) -> (110, -55)
  line L586 (140, -18) -> (149, -18)
  line L587 (149, -18) -> (149, -21)
  line L588 (149, -21) -> (154, -21)
  line L589 (140, -49) -> (149, -49)
  line L590 (149, -49) -> (149, -46)
  line L591 (149, -46) -> (154, -46)
  line L592 (154, -46) -> (154, -21)
  line L593 (140, -18) -> (140, -21)
  line L594 (140, -21) -> (135, -21)
  line L595 (135, -21) -> (135, -46)
  line L596 (135, -46) -> (140, -46)
  line L597 (140, -46) -> (140, -49)
  line L598 (118, -18) -> (127, -18)
  line L599 (127, -18) -> (127, -21)
  line L600 (127, -21) -> (132, -21)
  line L601 (132, -21) -> (132, -46)
  line L602 (132, -46) -> (127, -46)
  line L603 (127, -46) -> (127, -49)
  line L604 (127, -49) -> (118, -49)
  line L605 (118, -18) -> (118, -21)
  line L606 (118, -21) -> (113, -21)
  line L607 (113, -21) -> (113, -46)
  line L608 (113, -46) -> (118, -46)
  line L609 (118, -46) -> (118, -49)
  line L610 (96, -49) -> (105, -49)
  line L611 (105, -49) -> (105, -46)
  line L612 (105, -46) -> (110, -46)
  line L613 (110, -46) -> (110, -21)
  line L614 (96, -18) -> (96, -21)
  line L615 (96, -21) -> (91, -21)
  line L616 (91, -21) -> (91, -46)
  line L617 (91, -46) -> (96, -46)
  line L618 (96, -46) -> (96, -49)
  line L619 (96, -18) -> (105, -18)
  line L620 (105, -18) -> (105, -21)
  line L621 (105, -21) -> (110, -21)
  line L622 (63.1946, -126.4202) -> (45.6946, -126.4202)
  line L623 (45.6946, -126.4202) -> (45.6946, -129.4202)
  line L624 (45.6946, -129.4202) -> (36.6946, -129.4202)
  line L625 (36.6946, -129.4202) -> (36.6946, -126.4202)
  line L626 (36.6946, -126.4202) -> (31.6946, -126.4202)
  line L627 (31.6946, -126.4202) -> (31.6946, -101.4202)
  line L628 (31.6946, -101.4202) -> (36.6946, -101.4202)
  line L629 (36.6946, -101.4202) -> (36.6946, -98.4202)
  line L630 (36.6946, -98.4202) -> (45.6946, -98.4202)
  line L631 (120.241, 46) -> (110.241, 46)
  line L632 (110.241, 46) -> (110.241, 49)
  line L633 (110.241, 49) -> (100.241, 49)
  line L634 (100.241, 49) -> (100.241, 46)
  line L635 (100.241, 46) -> (90.241, 46)
  line L636 (90.241, 46) -> (90.241, 21)
  line L637 (90.241, 21) -> (100.241, 21)
  line L638 (100.241, 21) -> (100.241, 18)
  line L639 (100.241, 18) -> (110.241, 18)
  line L640 (110.241, 18) -> (110.241, 21)
  line L641 (110.241, 21) -> (120.241, 21)
  line L642 (120.241, 21) -> (120.241, 46)
  line L643 (153.241, 80) -> (143.241, 80)
  line L644 (143.241, 80) -> (143.241, 83)
  line L645 (143.241, 83) -> (133.241, 83)
  line L646 (133.241, 83) -> (133.241, 80)
  line L647 (133.241, 80) -> (123.241, 80)
  line L648 (123.241, 80) -> (123.241, 55)
  line L649 (123.241, 55) -> (133.241, 55)
  line L650 (133.241, 55) -> (133.241, 52)
  line L651 (133.241, 52) -> (143.241, 52)
  line L652 (143.241, 52) -> (143.241, 55)
  line L653 (143.241, 55) -> (153.241, 55)
  line L654 (153.241, 55) -> (153.241, 80)
  line L655 (120.241, 80) -> (110.241, 80)
  line L656 (110.241, 80) -> (110.241, 83)
  line L657 (110.241, 83) -> (100.241, 83)
  line L658 (100.241, 83) -> (100.241, 80)
  line L659 (100.241, 80) -> (90.241, 80)
  line L660 (90.241, 80) -> (90.241, 55)
  line L661 (90.241, 55) -> (100.241, 55)
  line L662 (100.241, 55) -> (100.241, 52)
  line L663 (100.241, 52) -> (110.241, 52)
  line L664 (110.241, 52) -> (110.241, 55)
  line L665 (110.241, 55) -> (120.241, 55)
  line L666 (120.241, 55) -> (120.241, 80)
  line L667 (-97, 46) -> (-97, 23)
  arc A0 (-102, 18) -> (-97, 23) centre (-102, 23) ccw
  line L668 (-102, 18) -> (-107, 18)
  arc A1 (-112, 23) -> (-107, 18) centre (-107, 23) ccw
  line L669 (-112, 23) -> (-112, 46)
  line L670 (-97, 82) -> (-92, 82)
  arc A2 (-92, 82) -> (-97, 87) centre (-97, 82) ccw
  line L671 (-97, 87) -> (-112, 87)
  arc A3 (-112, 87) -> (-117, 82) centre (-112, 82) ccw
  line L672 (-97, 82) -> (-97, 59)
  arc A4 (-102, 54) -> (-97, 59) centre (-102, 59) ccw
  line L673 (-102, 54) -> (-107, 54)
  arc A5 (-112, 59) -> (-107, 54) centre (-107, 59) ccw
  line L674 (-112, 59) -> (-112, 82)
  line L675 (-97, 46) -> (-92, 46)
  arc A6 (-92, 46) -> (-97, 51) centre (-97, 46) ccw
  line L676 (-97, 51) -> (-112, 51)
  arc A7 (-112, 51) -> (-117, 46) centre (-112, 46) ccw
  line L677 (-312.9327, 9.6476) -> (-312.9327, 6.6476)
  line L678 (-312.9327, 6.6476) -> (-322.9327, 6.6476)
  line L679 (-322.9327, 6.6476) -> (-322.9327, 9.6476)
  line L680 (63.1946, -126.4202) -> (63.1946, -129.4202)
  line L681 (63.1946, -129.4202) -> (69.1946, -129.4202)
  line L682 (69.1946, -98.4202) -> (63.1946, -98.4202)
  line L683 (63.1946, -98.4202) -> (63.1946, -101.4202)
  line L684 (63.1946, -101.4202) -> (45.6946, -101.4202)
  line L685 (-408.4327, -56.749) -> (-408.4327, -59.749)
  line L686 (-408.4327, -59.749) -> (-408.4327, -62.749)
  line L687 (-405.4327, -62.749) -> (-405.4327, -56.749)
  line L688 (-405.4327, -56.749) -> (-408.4327, -56.749)
  line L689 (-408.4327, -56.749) -> (-408.4327, -59.749)
  line L690 (-408.4327, -59.749) -> (-408.4327, -62.749)
  line L691 (-112, -66.5) -> (-112, -89.5)
  arc A8 (-112, -89.5) -> (-107, -94.5) centre (-107, -89.5) ccw
  line L692 (-107, -94.5) -> (-102, -94.5)
  arc A9 (-102, -94.5) -> (-97, -89.5) centre (-102, -89.5) ccw
  line L693 (-97, -89.5) -> (-97, -66.5)
  line L694 (-97, -66.5) -> (-92, -66.5)
  arc A10 (-92, -66.5) -> (-97, -61.5) centre (-97, -66.5) ccw
  line L695 (-97, -61.5) -> (-112, -61.5)
  arc A11 (-112, -61.5) -> (-117, -66.5) centre (-112, -66.5) ccw
  line L696 (-112, -30.5) -> (-112, -53.5)
  arc A12 (-112, -53.5) -> (-107, -58.5) centre (-107, -53.5) ccw
  line L697 (-107, -58.5) -> (-102, -58.5)
  arc A13 (-102, -58.5) -> (-97, -53.5) centre (-102, -53.5) ccw
  line L698 (-97, -53.5) -> (-97, -30.5)
  line L699 (-97, -30.5) -> (-92, -30.5)
  arc A14 (-92, -30.5) -> (-97, -25.5) centre (-97, -30.5) ccw
  line L700 (-97, -25.5) -> (-112, -25.5)
  arc A15 (-112, -25.5) -> (-117, -30.5) centre (-112, -30.5) ccw
  circle A16 centre (380, 118.5) radius 9
  circle A17 centre (198, 118.5) radius 9
  line L701 (304, -95) -> (304, -131)
  line L702 (274, -131) -> (274, -95)
  line L703 (168, 15) -> (168, -15)
  line L704 (168, 15) -> (204, 15)
  line L705 (410, 15) -> (407, 15)
  line L706 (407, 15) -> (404, 15)
  line L707 (274, -131) -> (304, -131)
  line L708 (160, -49) -> (163, -49)
  line L709 (163, -49) -> (163, -18)
  line L710 (163, -18) -> (198, -18)
  line L711 (201, -61) -> (201, -49)
  line L712 (201, -49) -> (198, -49)
  line L713 (198, -49) -> (198, -18)
  line L714 (204, 15) -> (198, 15)
  line L715 (274, -95) -> (268, -95)
  line L716 (304, -95) -> (310, -95)
  line L717 (268, 136) -> (268, 101)
  circle A18 centre (187, -61) radius 6.25
  circle A19 centre (391, -61) radius 6.25
  circle A20 centre (391, 61) radius 6.25
  circle A21 centre (187, 61) radius 6.25
  line L718 (143, -86) -> (140, -86)
  line L719 (252, -98) -> (252, -101)
  line L720 (268, -101) -> (268, -136)
  line L721 (252, -101) -> (268, -101)
  circle A22 centre (380, -118.5) radius 9
  circle A23 centre (198, -118.5) radius 9
  line L722 (160, -53.5) -> (160, -49)
  line L723 (201, -61) -> (201, -56.5)
  line L724 (418, -53.5) -> (418, -49)
  line L725 (418, 56.5) -> (418, 61)
  line L726 (160, 61) -> (160, 56.5)
  line L727 (252, -98) -> (243, -98)
  line L728 (329, 98) -> (326, 98)
  line L729 (246, 98) -> (243, 98)
  line L730 (246, -98) -> (243, -98)
  line L731 (329, -98) -> (326, -98)
  circle A24 centre (138.7318, -0.0139) radius 5
  line L732 (99, -86) -> (96, -86)
  line L733 (96, -117) -> (99, -117)
  line L734 (143, -52) -> (140, -52)
  line L735 (140, -83) -> (143, -83)
  line L736 (121, -52) -> (118, -52)
  line L737 (118, -83) -> (121, -83)
  line L738 (96, -83) -> (99, -83)
  line L739 (99, -52) -> (96, -52)
  line L740 (143, -18) -> (140, -18)
  line L741 (140, -49) -> (143, -49)
  line L742 (121, -18) -> (118, -18)
  line L743 (118, -49) -> (121, -49)
  line L744 (96, -49) -> (99, -49)
  line L745 (99, -18) -> (96, -18)
  line L746 (42.6946, -98.4202) -> (45.6946, -98.4202)
  line L747 (-102, 18) -> (-107, 18)
  circle A25 centre (-104.5, 40.5) radius 1.5
  circle A26 centre (-104.5, 23.5) radius 1.5
  circle A27 centre (-104.5, 76.5) radius 1.5
  line L748 (-117, 82) -> (-112, 82)
  circle A28 centre (-104.5, 59.5) radius 1.5
  line L749 (-117, 46) -> (-112, 46)
  line L750 (63.1946, -101.4202) -> (45.6946, -101.4202)
  line L751 (45.6946, -126.4202) -> (63.1946, -126.4202)
  line L752 (63.1946, -126.4202) -> (59.9446, -126.4202)
  circle A29 centre (-330.4327, -34.749) radius 1.5
  circle A30 centre (-380.4327, -34.749) radius 1.5
  line L753 (-405.4327, -62.749) -> (-408.4327, -62.749)
  line L754 (-405.4327, -62.749) -> (-405.4327, -56.749)
  line L755 (-405.4327, -6.749) -> (-408.4327, -6.749)
  circle A31 centre (-104.5, -89) radius 1.5
  line L756 (-117, -66.5) -> (-112, -66.5)
  circle A32 centre (-104.5, -53) radius 1.5
  circle A33 centre (-104.5, -36) radius 1.5
  line L757 (-117, -30.5) -> (-112, -30.5)
  circle A34 centre (-104.5, -72) radius 1.5
  line L758 (-102, -94.5) -> (-107, -94.5)
  line L759 (69.1946, -126.4202) -> (72.1946, -126.4202)
  line L760 (72.1946, -126.4202) -> (72.1946, -101.4202)
  line L761 (72.1946, -101.4202) -> (69.1946, -101.4202)
  line L762 (69.1946, -129.4202) -> (69.1946, -126.4202)
  line L763 (69.1946, -101.4202) -> (69.1946, -98.4202)
  line L764 (69.1946, -129.4202) -> (69.1946, -126.4202)
  line L765 (69.1946, -101.4202) -> (69.1946, -98.4202)
  line L766 (-405.4327, 15.6476) -> (-405.4327, 6.6476)
  line L767 (-408.4327, 15.6476) -> (-408.4327, 6.6476)
  line L768 (5, -125) -> (5, -128)
  line L769 (10, -125) -> (5, -125)
  line L770 (10, -128) -> (10, -125)
  line L771 (5, -128) -> (10, -128)
  line L772 (-5, -128) -> (-5, -125)
  line L773 (-5, -125) -> (-10, -125)
  line L774 (-10, -125) -> (-10, -128)
  line L775 (-10, -128) -> (-5, -128)
  circle A35 centre (0, -68) radius 3.75
  line L776 (15, -131) -> (-15, -131)
  line L777 (-15, -131) -> (-15, -95)
  line L778 (15, -95) -> (15, -131)
  line L779 (18, -9.875) -> (18, -6.875)
  line L780 (18, -6.875) -> (0, -6.875)
  line L781 (0, -9.875) -> (18, -9.875)
  line L782 (0, -6.875) -> (0, -9.875)
  line L783 (-5.25, -2) -> (-5.25, 2)
  line L784 (-9.25, 2) -> (-9.25, -2)
  line L785 (-9.25, -2) -> (-5.25, -2)
  line L786 (-5.25, 2) -> (-9.25, 2)
  line L787 (14.5, 35) -> (14.5, 25)
  line L788 (14.5, 25) -> (11.5, 25)
  line L789 (11.5, 25) -> (11.5, 35)
  line L790 (11.5, 35) -> (14.5, 35)
  line L791 (0, 59.125) -> (18, 59.125)
  line L792 (18, 62.125) -> (0, 62.125)
  line L793 (18, 59.125) -> (18, 62.125)
  line L794 (-11.5, 35) -> (-11.5, 25)
  line L795 (-11.5, 25) -> (-14.5, 25)
  line L796 (0, 62.125) -> (0, 59.125)
  circle A36 centre (0, 68) radius 3.75
  line L797 (-14.5, 35) -> (-11.5, 35)
  line L798 (-14.5, 25) -> (-14.5, 35)
  line L799 (20, 105.5) -> (20, 108.5)
  line L800 (5, 128) -> (5, 125)
  line L801 (15, 111.5) -> (15, 131)
  line L802 (10, 125) -> (10, 128)
  line L803 (5, 125) -> (10, 125)
  line L804 (10, 128) -> (5, 128)
  line L805 (15, 131) -> (-15, 131)
  line L806 (-5, 125) -> (-5, 128)
  line L807 (-5, 128) -> (-10, 128)
  line L808 (-10, 125) -> (-5, 125)
  line L809 (-10, 128) -> (-10, 125)
  line L810 (-15, 131) -> (-15, 95)
  line L811 (40, 92) -> (31, 92)
  line L812 (31, 92) -> (31, 89)
  line L813 (31, 89) -> (40, 89)
  line L814 (40, 89) -> (40, 92)
  line L815 (37, 82.5) -> (37, 85.5)
  line L816 (37, 85.5) -> (27, 85.5)
  line L817 (27, 85.5) -> (27, 82.5)
  line L818 (27, 82.5) -> (37, 82.5)
  line L819 (56, 85.5) -> (56, 70.5)
  line L820 (52.5, 108.5) -> (43.5, 108.5)
  line L821 (26, 108.5) -> (26, 105.5)
  line L822 (26, 105.5) -> (20, 105.5)
  line L823 (43.5, 108.5) -> (43.5, 105.5)
  line L824 (20, 108.5) -> (26, 108.5)
  line L825 (56, 111.5) -> (15, 111.5)
  line L826 (43.5, 105.5) -> (52.5, 105.5)
  line L827 (52.5, 105.5) -> (52.5, 108.5)
  line L828 (56, 95) -> (56, 111.5)
  line L829 (27, -22.5) -> (27, -25.5)
  line L830 (27, -25.5) -> (37, -25.5)
  line L831 (37, -25.5) -> (37, -22.5)
  line L832 (37, -22.5) -> (27, -22.5)
  line L833 (60.0916, -22) -> (60.0916, -26)
  line L834 (56.0916, -22) -> (60.0916, -22)
  line L835 (60.0916, -26) -> (56.0916, -26)
  line L836 (56, -26) -> (56, -22)
  line L837 (59, -70.5) -> (59, -85.5)
  line L838 (59, -85.5) -> (56, -85.5)
  line L839 (56, -85.5) -> (56, -70.5)
  line L840 (56, -70.5) -> (59, -70.5)
  line L841 (40, -92) -> (31, -92)
  line L842 (31, -92) -> (31, -89)
  line L843 (31, -89) -> (40, -89)
  line L844 (85, -95) -> (15, -95)
  line L845 (40, -89) -> (40, -92)
  line L846 (82, -24) -> (79, -24)
  line L847 (82, -24) -> (79, -24)
  line L848 (85, -37) -> (85, -15)
  line L849 (82, -15) -> (82, -24)
  line L850 (79, -15) -> (82, -15)
  line L851 (79, -24) -> (79, -15)
  line L852 (49.5, 35) -> (52.5, 35)
  line L853 (49.5, 25) -> (49.5, 35)
  line L854 (52.5, 25) -> (49.5, 25)
  line L855 (52.5, 35) -> (52.5, 25)
  circle A37 centre (58, 0) radius 3.75
  line L856 (79, -80) -> (79, -89)
  line L857 (79, -89) -> (82, -89)
  line L858 (82, -89) -> (82, -80)
  line L859 (82, -80) -> (79, -80)
  line L860 (85, -15) -> (85, -95)
  line L861 (79, -46) -> (82, -46)
  line L862 (79, -58) -> (79, -46)
  line L863 (82, -58) -> (79, -58)
  line L864 (82, -46) -> (82, -58)
  line L865 (82, 15) -> (82, 24)
  line L866 (79, 24) -> (79, 15)
  line L867 (82, 24) -> (79, 24)
  line L868 (121, 15) -> (85, 15)
  line L869 (56, 70.5) -> (59, 70.5)
  line L870 (59, 70.5) -> (59, 85.5)
  line L871 (59, 85.5) -> (56, 85.5)
  line L872 (82, 89) -> (82, 80)
  line L873 (82, 80) -> (79, 80)
  line L874 (85, 95) -> (56, 95)
  line L875 (79, 80) -> (79, 89)
  line L876 (82, 58) -> (79, 58)
  line L877 (85, 15) -> (85, 95)
  line L878 (82, 46) -> (82, 58)
  line L879 (79, 58) -> (79, 46)
  line L880 (79, 46) -> (82, 46)
  line L881 (85, -15) -> (121, -15)
  line L882 (82, 80) -> (79, 80)
  line L883 (79, 89) -> (82, 89)
  line L884 (82, 15) -> (79, 15)
  line L885 (79, -89) -> (82, -89)
  line L886 (115, 5) -> (118, 5)
  line L887 (118, 5) -> (118, 10)
  line L888 (118, 10) -> (115, 10)
  line L889 (115, 10) -> (115, 5)
  line L890 (118, -5) -> (115, -5)
  line L891 (118, -10) -> (118, -5)
  line L892 (115, -10) -> (118, -10)
  line L893 (115, -5) -> (115, -10)
  line L894 (-79, -89) -> (-79, -80)
  line L895 (-79, -80) -> (-82, -80)
  line L896 (-82, -89) -> (-79, -89)
  line L897 (-82, -80) -> (-82, -89)
  line L898 (-31, -92) -> (-40, -92)
  line L899 (-40, -92) -> (-40, -89)
  line L900 (-31, -89) -> (-31, -92)
  line L901 (-40, -89) -> (-31, -89)
  line L902 (-27, -25.5) -> (-37, -25.5)
  line L903 (-37, -25.5) -> (-37, -22.5)
  line L904 (-37, -22.5) -> (-27, -22.5)
  line L905 (-60, -26) -> (-60, -22)
  circle A38 centre (-58, 0) radius 3.75
  line L906 (-60, -22) -> (-56, -22)
  line L907 (-56, -22) -> (-56, -26)
  line L908 (-56, -26) -> (-60, -26)
  line L909 (-27, -22.5) -> (-27, -25.5)
  line L910 (-82, -46) -> (-79, -46)
  line L911 (-79, -46) -> (-79, -58)
  line L912 (-79, -58) -> (-82, -58)
  line L913 (-82, -58) -> (-82, -46)
  line L914 (-79, -15) -> (-79, -24)
  line L915 (-79, -24) -> (-82, -24)
  line L916 (-82, -24) -> (-82, -15)
  line L917 (-79, -24) -> (-82, -24)
  line L918 (-82, -15) -> (-79, -15)
  line L919 (-59, -70.5) -> (-59, -85.5)
  line L920 (-59, -85.5) -> (-56, -85.5)
  line L921 (-15, -95) -> (-85, -95)
  line L922 (-56, -85.5) -> (-56, -70.5)
  line L923 (-56, -70.5) -> (-59, -70.5)
  line L924 (-49.5, 35) -> (-52.5, 35)
  line L925 (-49.5, 25) -> (-49.5, 35)
  line L926 (-52.5, 25) -> (-49.5, 25)
  line L927 (-52.5, 35) -> (-52.5, 25)
  line L928 (-56, 70.5) -> (-59, 70.5)
  line L929 (-59, 70.5) -> (-59, 85.5)
  line L930 (-79, 46) -> (-82, 46)
  line L931 (-79, 58) -> (-79, 46)
  line L932 (-82, 58) -> (-79, 58)
  line L933 (-82, 46) -> (-82, 58)
  line L934 (-85, 95) -> (-85, 15)
  line L935 (-56, 85.5) -> (-56, 70.5)
  line L936 (-59, 85.5) -> (-56, 85.5)
  line L937 (-15, 95) -> (-85, 95)
  line L938 (-31, 89) -> (-31, 92)
  line L939 (-37, 82.5) -> (-37, 85.5)
  line L940 (-27, 82.5) -> (-37, 82.5)
  line L941 (-27, 85.5) -> (-27, 82.5)
  line L942 (-37, 85.5) -> (-27, 85.5)
  line L943 (-82, 24) -> (-79, 24)
  line L944 (-79, 24) -> (-79, 15)
  line L945 (-79, 15) -> (-82, 15)
  line L946 (-82, 15) -> (-82, 24)
  line L947 (-79, 89) -> (-79, 80)
  line L948 (-82, 89) -> (-79, 89)
  line L949 (-82, 80) -> (-82, 89)
  line L950 (-79, 80) -> (-82, 80)
  line L951 (-79, 80) -> (-82, 80)
  line L952 (-40, 92) -> (-40, 89)
  line L953 (-31, 92) -> (-40, 92)
  line L954 (-40, 89) -> (-31, 89)
  line L955 (-79, -89) -> (-82, -89)
  line L956 (-85, -15) -> (-121, -15)
  line L957 (-85, -95) -> (-85, -15)
  line L958 (-85, 15) -> (-121, 15)
  line L959 (-115, -5) -> (-115, -10)
  line L960 (-115, -10) -> (-118, -10)
  line L961 (-118, -10) -> (-118, -5)
  line L962 (-118, -5) -> (-115, -5)
  line L963 (-115, 10) -> (-115, 5)
  line L964 (-115, 5) -> (-118, 5)
  line L965 (-118, 5) -> (-118, 10)
  line L966 (-118, 10) -> (-115, 10)
  line L967 (121, 15) -> (121, -15)
  line L968 (-153, 111.5) -> (-153, 95)
  line L969 (-153, 111.5) -> (-153, 95)
  line L970 (-153, 95) -> (-153, 111.5)
  line L971 (-156.5, 105.5) -> (-156.5, 108.5)
  line L972 (-165.5, 105.5) -> (-156.5, 105.5)
  line L973 (-156.5, 108.5) -> (-165.5, 108.5)
  line L974 (-165.5, 108.5) -> (-165.5, 105.5)
  line L975 (-194, 111.5) -> (-153, 111.5)
  line L976 (-153, 111.5) -> (-194, 111.5)
  line L977 (-194, 111.5) -> (-153, 111.5)
  line L978 (-183, 108.5) -> (-189, 108.5)
  line L979 (-194, 95) -> (-194, 111.5)
  line L980 (-183, 105.5) -> (-183, 108.5)
  line L981 (-189, 105.5) -> (-183, 105.5)
  line L982 (-189, 108.5) -> (-189, 105.5)
  line L983 (-194, 95) -> (-194, 111.5)
  line L984 (-294, 95) -> (-194, 95)
  line L985 (-191, 62.125) -> (-191, 59.125)
  circle A39 centre (-209, 68) radius 3.75
  circle A40 centre (-229, 53.0625) radius 1.5
  line L986 (-209, 59.125) -> (-209, 62.125)
  line L987 (-209, 62.125) -> (-191, 62.125)
  circle A41 centre (-189, 53.0625) radius 1.5
  line L988 (-191, 59.125) -> (-209, 59.125)
  line L989 (-294, -95) -> (-294, 95)
  line L990 (-294, -95) -> (-294, 95)
  line L991 (-294, 15) -> (-294, 95)
  line L992 (-288, -80) -> (-291, -80)
  line L993 (-291, -80) -> (-291, -89)
  line L994 (-291, -89) -> (-288, -89)
  line L995 (-288, -89) -> (-288, -80)
  line L996 (-130, -80) -> (-130, -89)
  circle A42 centre (-209, -68) radius 3.75
  line L997 (-130, -89) -> (-127, -89)
  line L998 (-127, -89) -> (-127, -80)
  line L999 (-127, -80) -> (-130, -80)
  line L1000 (-194, 111.5) -> (-194, 95)
  line L1001 (-246, 85.5) -> (-236, 85.5)
  circle A43 centre (-209, 89.5) radius 2.5
  line L1002 (-236, 85.5) -> (-236, 82.5)
  line L1003 (-246, 82.5) -> (-246, 85.5)
  line L1004 (-236, 82.5) -> (-246, 82.5)
  line L1005 (-194, 95) -> (-294, 95)
  line L1006 (-294, 95) -> (-194, 95)
  line L1007 (-172, 85.5) -> (-182, 85.5)
  line L1008 (-182, 85.5) -> (-182, 82.5)
  line L1009 (-182, 82.5) -> (-172, 82.5)
  line L1010 (-172, 82.5) -> (-172, 85.5)
  line L1011 (-288, 80) -> (-291, 80)
  line L1012 (-288, 89) -> (-288, 80)
  line L1013 (-291, 80) -> (-291, 89)
  line L1014 (-288, 80) -> (-291, 80)
  line L1015 (-291, 89) -> (-288, 89)
  line L1016 (-153, 95) -> (-124, 95)
  line L1017 (-127, 89) -> (-127, 80)
  line L1018 (-127, 80) -> (-130, 80)
  line L1019 (-130, 80) -> (-130, 89)
  line L1020 (-127, 80) -> (-130, 80)
  line L1021 (-130, 89) -> (-127, 89)
  line L1022 (-153, 95) -> (-124, 95)
  circle A44 centre (-229, 8.0625) radius 1.5
  line L1023 (-220.5, 25) -> (-223.5, 25)
  circle A45 centre (-249, 19.5) radius 1.5
  line L1024 (-220.5, 35) -> (-220.5, 25)
  line L1025 (-223.5, 35) -> (-220.5, 35)
  line L1026 (-223.5, 25) -> (-223.5, 35)
  line L1027 (-159.5, 25) -> (-156.5, 25)
  line L1028 (-156.5, 35) -> (-159.5, 35)
  line L1029 (-159.5, 35) -> (-159.5, 25)
  line L1030 (-156.5, 25) -> (-156.5, 35)
  circle A46 centre (-145, 19.5) radius 1.5
  line L1031 (-214.25, 2) -> (-218.25, 2)
  line L1032 (-218.25, 2) -> (-218.25, -2)
  line L1033 (-214.25, -2) -> (-214.25, 2)
  line L1034 (-218.25, -2) -> (-214.25, -2)
  line L1035 (-209, -9.875) -> (-209, -6.875)
  line L1036 (-241.5, -5) -> (-241.5, -2)
  line L1037 (-241.5, -2) -> (-251.5, -2)
  line L1038 (-251.5, -2) -> (-251.5, -5)
  line L1039 (-251.5, -5) -> (-241.5, -5)
  line L1040 (-262, -8) -> (-259, -8)
  line L1041 (-262, -2) -> (-262, -8)
  line L1042 (-259, -2) -> (-262, -2)
  circle A47 centre (-267, 0) radius 3.75
  line L1043 (-259, -8) -> (-259, -2)
  line L1044 (-261.5, 35) -> (-258.5, 35)
  line L1045 (-258.5, 35) -> (-258.5, 25)
  line L1046 (-258.5, 25) -> (-261.5, 25)
  line L1047 (-261.5, 25) -> (-261.5, 35)
  circle A48 centre (-273, 19.5) radius 1.5
  line L1048 (-176.5, -5) -> (-176.5, -2)
  line L1049 (-176.5, -2) -> (-166.5, -2)
  line L1050 (-166.5, -2) -> (-166.5, -5)
  circle A49 centre (-151, 0) radius 3.75
  line L1051 (-159, -2) -> (-156, -2)
  line L1052 (-156, -2) -> (-156, -8)
  line L1053 (-156, -8) -> (-159, -8)
  line L1054 (-159, -8) -> (-159, -2)
  line L1055 (-166.5, -5) -> (-176.5, -5)
  circle A50 centre (-169, 19.5) radius 1.5
  line L1056 (-262, -34.5) -> (-259, -34.5)
  line L1057 (-259, -25.5) -> (-262, -25.5)
  line L1058 (-262, -25.5) -> (-262, -34.5)
  line L1059 (-259, -34.5) -> (-259, -25.5)
  line L1060 (-246, -25.5) -> (-246, -22.5)
  line L1061 (-246, -22.5) -> (-236, -22.5)